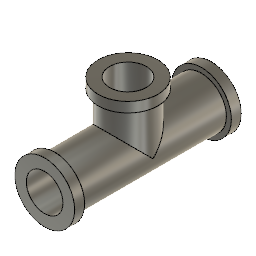
Semana4_Desafio3 v1 (Autodesk Fusion 360 design; units mm, degrees)
Autodesk Fusion 360 part; units mm, degrees
note: some values were not read from the file. Set by a fixed rule: which sketch regions a step uses.
sketch "Sketch6" plane through (0, 0, 0) normal (1, 0, 0) x (0, 1, 0)
  line L0 (-25, 0) -> (25, 0)
  dimension "d9" = 50
  constraint horizontal L0
  measures "d9" distance of L0.start L0.end
pipe "Pipe2" add diameter 15 wall 2 path "Sketch6" along L0
sketch "Sketch8" plane through (0, 0, 0) normal (1, 0, 0) x (0, 1, 0)
  line L0 (0, 0) -> (0, 17.5)
  dimension "d15" = 17.5
  constraint coincident L0.start origin
  constraint vertical L0
  measures "d15" distance of L0.start L0.end
pipe "Pipe3" add diameter 15 wall 2 path "Sketch8" along L0
sketch "Sketch9" plane through (0, 0, 0) normal (0, 1, 0) x (1, 0, 0)
  circle A0 centre (0, 0) radius 5.5
  dimension "d20" = 11
  constraint coincident A0.centre origin
  measures "d20" diameter of A0
extrude "Extrude1" cut sketch "Sketch9" along normal mid plane 236
sketch "Sketch10" plane through (0, 0, 0) normal (0, 0, 1) x (1, 0, 0)
  circle A0 centre (0, 0) radius 5.5
  dimension "d23" = 11
  constraint coincident A0.centre origin
  measures "d23" diameter of A0
extrude "Extrude2" cut sketch "Sketch10" along normal blind 27
ref_plane "WorkPlane2" through (0, 25, 0) normal (0, 1, 0) x (0, 0, 1)
sketch "Sketch11" plane through (0, 25, 0) normal (0, 1, 0) x (1, 0, 0)
  circle A0 centre (0, 0) radius 7.5
  circle A1 centre (0, 0) radius 9
  dimension "d27" = 15
  constraint coincident A0.centre A1.centre
  measures "d27" diameter of A0
extrude "Extrude3" add sketch "Sketch11" against normal blind 3
ref_plane "WorkPlane3" through (0, -25, 0) normal (0, 1, 0) x (0, 0, 1)
sketch "Sketch12" plane through (0, -25, 0) normal (0, 1, 0) x (1, 0, 0)
  circle A0 centre (0, 0) radius 9
  circle A1 centre (0, 0) radius 7.5
  dimension "d31" = 15
  constraint coincident A0.centre A1.centre
  constraint concentric A0 A1
  measures "d31" diameter of A1
extrude "Extrude4" add sketch "Sketch12" along normal blind 3
ref_plane "WorkPlane4" through (0, 0, 17.5) normal (0, 0, 1) x (1, 0, 0)
sketch "Sketch13" plane through (0, 0, 17.5) normal (0, 0, 1) x (1, 0, 0)
  circle A0 centre (0, 0) radius 9
  circle A1 centre (0, 0) radius 7.5
  dimension "d35" = 18
  dimension "d36" = 15
  constraint coincident A0.centre A1.centre
  measures "d35" diameter of A0
  measures "d36" diameter of A1
extrude "Extrude5" add sketch "Sketch13" against normal blind 3
